Autodesk Fusion 360 part; units mm, degrees
(part 7 of 9)
sketch "Sketch13" plane through (0, 0.6, 0) normal (0, -1, 0) x (1, 0, 0)
  circle A0 centre (32.525, 66.675) radius 2
  circle A1 centre (245.269, 9.525) radius 2
  circle A2 centre (47.625, 9.525) radius 2
  circle A3 centre (220.025, 66.675) radius 2
  circle A4 centre (128.588, 37.025) radius 2
  arc A5 (94.0125, 35.575) -> (93.0125, 34.575) centre (94.0125, 34.575) ccw
  line L0 (94.0125, 35.575) -> (106.0125, 35.575)
  arc A6 (107.0125, 34.575) -> (106.0125, 35.575) centre (106.0125, 34.575) ccw
  line L1 (107.0125, 34.575) -> (107.0125, 22.575)
  arc A7 (106.0125, 21.575) -> (107.0125, 22.575) centre (106.0125, 22.575) ccw
  line L2 (106.0125, 21.575) -> (94.0125, 21.575)
  arc A8 (93.0125, 22.575) -> (94.0125, 21.575) centre (94.0125, 22.575) ccw
  line L3 (93.0125, 22.575) -> (93.0125, 34.575)
  arc A9 (132.1125, 35.575) -> (131.1125, 34.575) centre (132.1125, 34.575) ccw
  line L4 (132.1125, 35.575) -> (144.1125, 35.575)
  arc A10 (145.1125, 34.575) -> (144.1125, 35.575) centre (144.1125, 34.575) ccw
  line L5 (145.1125, 34.575) -> (145.1125, 22.575)
  arc A11 (144.1125, 21.575) -> (145.1125, 22.575) centre (144.1125, 22.575) ccw
  line L6 (144.1125, 21.575) -> (132.1125, 21.575)
  arc A12 (131.1125, 22.575) -> (132.1125, 21.575) centre (132.1125, 22.575) ccw
  line L7 (131.1125, 22.575) -> (131.1125, 34.575)
  arc A13 (251.175, 16.525) -> (250.175, 15.525) centre (251.175, 15.525) ccw
  line L8 (251.175, 16.525) -> (263.175, 16.525)
  arc A14 (264.175, 15.525) -> (263.175, 16.525) centre (263.175, 15.525) ccw
  line L9 (264.175, 15.525) -> (264.175, 3.525)
  arc A15 (263.175, 2.525) -> (264.175, 3.525) centre (263.175, 3.525) ccw
  line L10 (263.175, 2.525) -> (251.175, 2.525)
  arc A16 (250.175, 3.525) -> (251.175, 2.525) centre (251.175, 3.525) ccw
  line L11 (250.175, 3.525) -> (250.175, 15.525)
  arc A17 (217.8375, 54.625) -> (216.8375, 53.625) centre (217.8375, 53.625) ccw
  line L12 (217.8375, 54.625) -> (229.8375, 54.625)
  arc A18 (230.8375, 53.625) -> (229.8375, 54.625) centre (229.8375, 53.625) ccw
  line L13 (230.8375, 53.625) -> (230.8375, 41.625)
  arc A19 (229.8375, 40.625) -> (230.8375, 41.625) centre (229.8375, 41.625) ccw
  line L14 (229.8375, 40.625) -> (217.8375, 40.625)
  arc A20 (216.8375, 41.625) -> (217.8375, 40.625) centre (217.8375, 41.625) ccw
  line L15 (216.8375, 41.625) -> (216.8375, 53.625)
  arc A21 (179.7375, 54.625) -> (178.7375, 53.625) centre (179.7375, 53.625) ccw
  line L16 (179.7375, 54.625) -> (191.7375, 54.625)
  arc A22 (192.7375, 53.625) -> (191.7375, 54.625) centre (191.7375, 53.625) ccw
  line L17 (192.7375, 53.625) -> (192.7375, 41.625)
  arc A23 (191.7375, 40.625) -> (192.7375, 41.625) centre (191.7375, 41.625) ccw
  line L18 (191.7375, 40.625) -> (179.7375, 40.625)
  arc A24 (178.7375, 41.625) -> (179.7375, 40.625) centre (179.7375, 41.625) ccw
  line L19 (178.7375, 41.625) -> (178.7375, 53.625)
  arc A25 (108.3, 16.525) -> (107.3, 15.525) centre (108.3, 15.525) ccw
  line L20 (108.3, 16.525) -> (120.3, 16.525)
  arc A26 (121.3, 15.525) -> (120.3, 16.525) centre (120.3, 15.525) ccw
  line L21 (121.3, 15.525) -> (121.3, 3.525)
  arc A27 (120.3, 2.525) -> (121.3, 3.525) centre (120.3, 3.525) ccw
  line L22 (120.3, 2.525) -> (108.3, 2.525)
  arc A28 (107.3, 3.525) -> (108.3, 2.525) centre (108.3, 3.525) ccw
  line L23 (107.3, 3.525) -> (107.3, 15.525)
  arc A29 (203.55, 16.525) -> (202.55, 15.525) centre (203.55, 15.525) ccw
  line L24 (203.55, 16.525) -> (215.55, 16.525)
  arc A30 (216.55, 15.525) -> (215.55, 16.525) centre (215.55, 15.525) ccw
  line L25 (216.55, 15.525) -> (216.55, 3.525)
  arc A31 (215.55, 2.525) -> (216.55, 3.525) centre (215.55, 3.525) ccw
  line L26 (215.55, 2.525) -> (203.55, 2.525)
  arc A32 (202.55, 3.525) -> (203.55, 2.525) centre (203.55, 3.525) ccw
  line L27 (202.55, 3.525) -> (202.55, 15.525)
  arc A33 (189.2625, 35.575) -> (188.2625, 34.575) centre (189.2625, 34.575) ccw
  line L28 (189.2625, 35.575) -> (201.2625, 35.575)
  arc A34 (202.2625, 34.575) -> (201.2625, 35.575) centre (201.2625, 34.575) ccw
  line L29 (202.2625, 34.575) -> (202.2625, 22.575)
  arc A35 (201.2625, 21.575) -> (202.2625, 22.575) centre (201.2625, 22.575) ccw
  line L30 (201.2625, 21.575) -> (189.2625, 21.575)
  arc A36 (188.2625, 22.575) -> (189.2625, 21.575) centre (189.2625, 22.575) ccw
  line L31 (188.2625, 22.575) -> (188.2625, 34.575)
  arc A37 (146.4, 16.525) -> (145.4, 15.525) centre (146.4, 15.525) ccw
  line L32 (146.4, 16.525) -> (158.4, 16.525)
  arc A38 (159.4, 15.525) -> (158.4, 16.525) centre (158.4, 15.525) ccw
  line L33 (159.4, 15.525) -> (159.4, 3.525)
  arc A39 (158.4, 2.525) -> (159.4, 3.525) centre (158.4, 3.525) ccw
  line L34 (158.4, 2.525) -> (146.4, 2.525)
  arc A40 (145.4, 3.525) -> (146.4, 2.525) centre (146.4, 3.525) ccw
  line L35 (145.4, 3.525) -> (145.4, 15.525)
  arc A41 (113.0625, 35.575) -> (112.0625, 34.575) centre (113.0625, 34.575) ccw
  line L36 (113.0625, 35.575) -> (125.0625, 35.575)
  arc A42 (126.0625, 34.575) -> (125.0625, 35.575) centre (125.0625, 34.575) ccw
  line L37 (126.0625, 34.575) -> (126.0625, 22.575)
  arc A43 (125.0625, 21.575) -> (126.0625, 22.575) centre (125.0625, 22.575) ccw
  line L38 (125.0625, 21.575) -> (113.0625, 21.575)
  arc A44 (112.0625, 22.575) -> (113.0625, 21.575) centre (113.0625, 22.575) ccw
  line L39 (112.0625, 22.575) -> (112.0625, 34.575)
  arc A45 (127.35, 16.525) -> (126.35, 15.525) centre (127.35, 15.525) ccw
  line L40 (127.35, 16.525) -> (139.35, 16.525)
  arc A46 (140.35, 15.525) -> (139.35, 16.525) centre (139.35, 15.525) ccw
  line L41 (140.35, 15.525) -> (140.35, 3.525)
  arc A47 (139.35, 2.525) -> (140.35, 3.525) centre (139.35, 3.525) ccw
  line L42 (139.35, 2.525) -> (127.35, 2.525)
  arc A48 (126.35, 3.525) -> (127.35, 2.525) centre (127.35, 3.525) ccw
  line L43 (126.35, 3.525) -> (126.35, 15.525)
  arc A49 (170.2125, 35.575) -> (169.2125, 34.575) centre (170.2125, 34.575) ccw
  line L44 (170.2125, 35.575) -> (182.2125, 35.575)
  arc A50 (183.2125, 34.575) -> (182.2125, 35.575) centre (182.2125, 34.575) ccw
  line L45 (183.2125, 34.575) -> (183.2125, 22.575)
  arc A51 (182.2125, 21.575) -> (183.2125, 22.575) centre (182.2125, 22.575) ccw
  line L46 (182.2125, 21.575) -> (170.2125, 21.575)
  arc A52 (169.2125, 22.575) -> (170.2125, 21.575) centre (170.2125, 22.575) ccw
  line L47 (169.2125, 22.575) -> (169.2125, 34.575)
  arc A53 (224.9813, 73.675) -> (223.9813, 72.675) centre (224.9813, 72.675) ccw
  line L48 (224.9813, 73.675) -> (236.9813, 73.675)
  arc A54 (237.9812, 72.675) -> (236.9813, 73.675) centre (236.9813, 72.675) ccw
  line L49 (237.9812, 72.675) -> (237.9813, 60.675)
  arc A55 (236.9813, 59.675) -> (237.9813, 60.675) centre (236.9813, 60.675) ccw
  line L50 (236.9813, 59.675) -> (224.9813, 59.675)
  arc A56 (223.9812, 60.675) -> (224.9813, 59.675) centre (224.9813, 60.675) ccw
  line L51 (223.9812, 60.675) -> (223.9813, 72.675)
  arc A57 (198.7875, 54.625) -> (197.7875, 53.625) centre (198.7875, 53.625) ccw
  line L52 (198.7875, 54.625) -> (210.7875, 54.625)
  arc A58 (211.7875, 53.625) -> (210.7875, 54.625) centre (210.7875, 53.625) ccw
  line L53 (211.7875, 53.625) -> (211.7875, 41.625)
  arc A59 (210.7875, 40.625) -> (211.7875, 41.625) centre (210.7875, 41.625) ccw
  line L54 (210.7875, 40.625) -> (198.7875, 40.625)
  arc A60 (197.7875, 41.625) -> (198.7875, 40.625) centre (198.7875, 41.625) ccw
  line L55 (197.7875, 41.625) -> (197.7875, 53.625)
  arc A61 (51.15, 16.525) -> (50.15, 15.525) centre (51.15, 15.525) ccw
  line L56 (51.15, 16.525) -> (63.15, 16.525)
  arc A62 (64.15, 15.525) -> (63.15, 16.525) centre (63.15, 15.525) ccw
  line L57 (64.15, 15.525) -> (64.15, 3.525)
  arc A63 (63.15, 2.525) -> (64.15, 3.525) centre (63.15, 3.525) ccw
  line L58 (63.15, 2.525) -> (51.15, 2.525)
  arc A64 (50.15, 3.525) -> (51.15, 2.525) centre (51.15, 3.525) ccw
  line L59 (50.15, 3.525) -> (50.15, 15.525)
  arc A65 (8.2875, 16.525) -> (7.2875, 15.525) centre (8.2875, 15.525) ccw
  line L60 (8.2875, 16.525) -> (20.2875, 16.525)
  arc A66 (21.2875, 15.525) -> (20.2875, 16.525) centre (20.2875, 15.525) ccw
  line L61 (21.2875, 15.525) -> (21.2875, 3.525)
  arc A67 (20.2875, 2.525) -> (21.2875, 3.525) centre (20.2875, 3.525) ccw
  line L62 (20.2875, 2.525) -> (8.2875, 2.525)
  arc A68 (7.2875, 3.525) -> (8.2875, 2.525) centre (8.2875, 3.525) ccw
  line L63 (7.2875, 3.525) -> (7.2875, 15.525)
  arc A69 (208.3125, 35.575) -> (207.3125, 34.575) centre (208.3125, 34.575) ccw
  line L64 (208.3125, 35.575) -> (220.3125, 35.575)
  arc A70 (221.3125, 34.575) -> (220.3125, 35.575) centre (220.3125, 34.575) ccw
  line L65 (221.3125, 34.575) -> (221.3125, 22.575)
  arc A71 (220.3125, 21.575) -> (221.3125, 22.575) centre (220.3125, 22.575) ccw
  line L66 (220.3125, 21.575) -> (208.3125, 21.575)
  arc A72 (207.3125, 22.575) -> (208.3125, 21.575) centre (208.3125, 22.575) ccw
  line L67 (207.3125, 22.575) -> (207.3125, 34.575)
  arc A73 (227.3625, 16.525) -> (226.3625, 15.525) centre (227.3625, 15.525) ccw
  line L68 (227.3625, 16.525) -> (239.3625, 16.525)
  arc A74 (240.3625, 15.525) -> (239.3625, 16.525) centre (239.3625, 15.525) ccw
  line L69 (240.3625, 15.525) -> (240.3625, 3.525)
  arc A75 (239.3625, 2.525) -> (240.3625, 3.525) centre (239.3625, 3.525) ccw
  line L70 (239.3625, 2.525) -> (227.3625, 2.525)
  arc A76 (226.3625, 3.525) -> (227.3625, 2.525) centre (227.3625, 3.525) ccw
  line L71 (226.3625, 3.525) -> (226.3625, 15.525)
  arc A77 (74.9625, 35.575) -> (73.9625, 34.575) centre (74.9625, 34.575) ccw
  line L72 (74.9625, 35.575) -> (86.9625, 35.575)
  arc A78 (87.9625, 34.575) -> (86.9625, 35.575) centre (86.9625, 34.575) ccw
  line L73 (87.9625, 34.575) -> (87.9625, 22.575)
  arc A79 (86.9625, 21.575) -> (87.9625, 22.575) centre (86.9625, 22.575) ccw
  line L74 (86.9625, 21.575) -> (74.9625, 21.575)
  arc A80 (73.9625, 22.575) -> (74.9625, 21.575) centre (74.9625, 22.575) ccw
  line L75 (73.9625, 22.575) -> (73.9625, 34.575)
  arc A81 (41.625, 73.675) -> (40.625, 72.675) centre (41.625, 72.675) ccw
  line L76 (41.625, 73.675) -> (53.625, 73.675)
  arc A82 (54.625, 72.675) -> (53.625, 73.675) centre (53.625, 72.675) ccw
  line L77 (54.625, 72.675) -> (54.625, 60.675)
  arc A83 (53.625, 59.675) -> (54.625, 60.675) centre (53.625, 60.675) ccw
  line L78 (53.625, 59.675) -> (41.625, 59.675)
  arc A84 (40.625, 60.675) -> (41.625, 59.675) centre (41.625, 60.675) ccw
  line L79 (40.625, 60.675) -> (40.625, 72.675)
  arc A85 (89.25, 16.525) -> (88.25, 15.525) centre (89.25, 15.525) ccw
  line L80 (89.25, 16.525) -> (101.25, 16.525)
  arc A86 (102.25, 15.525) -> (101.25, 16.525) centre (101.25, 15.525) ccw
  line L81 (102.25, 15.525) -> (102.25, 3.525)
  arc A87 (101.25, 2.525) -> (102.25, 3.525) centre (101.25, 3.525) ccw
  line L82 (101.25, 2.525) -> (89.25, 2.525)
  arc A88 (88.25, 3.525) -> (89.25, 2.525) centre (89.25, 3.525) ccw
  line L83 (88.25, 3.525) -> (88.25, 15.525)
  arc A89 (151.1625, 35.575) -> (150.1625, 34.575) centre (151.1625, 34.575) ccw
  line L84 (151.1625, 35.575) -> (163.1625, 35.575)
  arc A90 (164.1625, 34.575) -> (163.1625, 35.575) centre (163.1625, 34.575) ccw
  line L85 (164.1625, 34.575) -> (164.1625, 22.575)
  arc A91 (163.1625, 21.575) -> (164.1625, 22.575) centre (163.1625, 22.575) ccw
  line L86 (163.1625, 21.575) -> (151.1625, 21.575)
  arc A92 (150.1625, 22.575) -> (151.1625, 21.575) centre (151.1625, 22.575) ccw
  line L87 (150.1625, 22.575) -> (150.1625, 34.575)
  arc A93 (172.5938, 73.675) -> (171.5938, 72.675) centre (172.5938, 72.675) ccw
  line L88 (172.5938, 73.675) -> (184.5938, 73.675)
  arc A94 (185.5937, 72.675) -> (184.5938, 73.675) centre (184.5937, 72.675) ccw
  line L89 (185.5937, 72.675) -> (185.5937, 60.675)
  arc A95 (184.5938, 59.675) -> (185.5937, 60.675) centre (184.5938, 60.675) ccw
  line L90 (184.5938, 59.675) -> (172.5937, 59.675)
  arc A96 (171.5938, 60.675) -> (172.5938, 59.675) centre (172.5938, 60.675) ccw
  line L91 (171.5937, 60.675) -> (171.5938, 72.675)
  arc A97 (70.2, 16.525) -> (69.2, 15.525) centre (70.2, 15.525) ccw
  line L92 (70.2, 16.525) -> (82.2, 16.525)
  arc A98 (83.2, 15.525) -> (82.2, 16.525) centre (82.2, 15.525) ccw
  line L93 (83.2, 15.525) -> (83.2, 3.525)
  arc A99 (82.2, 2.525) -> (83.2, 3.525) centre (82.2, 3.525) ccw
  line L94 (82.2, 2.525) -> (70.2, 2.525)
  arc A100 (69.2, 3.525) -> (70.2, 2.525) centre (70.2, 3.525) ccw
  line L95 (69.2, 3.525) -> (69.2, 15.525)
  arc A101 (46.3875, 54.625) -> (45.3875, 53.625) centre (46.3875, 53.625) ccw
  line L96 (46.3875, 54.625) -> (58.3875, 54.625)
  arc A102 (59.3875, 53.625) -> (58.3875, 54.625) centre (58.3875, 53.625) ccw
  line L97 (59.3875, 53.625) -> (59.3875, 41.625)
  arc A103 (58.3875, 40.625) -> (59.3875, 41.625) centre (58.3875, 41.625) ccw
  line L98 (58.3875, 40.625) -> (46.3875, 40.625)
  arc A104 (45.3875, 41.625) -> (46.3875, 40.625) centre (46.3875, 41.625) ccw
  line L99 (45.3875, 41.625) -> (45.3875, 53.625)
  arc A105 (55.9125, 35.575) -> (54.9125, 34.575) centre (55.9125, 34.575) ccw
  line L100 (55.9125, 35.575) -> (67.9125, 35.575)
  arc A106 (68.9125, 34.575) -> (67.9125, 35.575) centre (67.9125, 34.575) ccw
  line L101 (68.9125, 34.575) -> (68.9125, 22.575)
  arc A107 (67.9125, 21.575) -> (68.9125, 22.575) centre (67.9125, 22.575) ccw
  line L102 (67.9125, 21.575) -> (55.9125, 21.575)
  arc A108 (54.9125, 22.575) -> (55.9125, 21.575) centre (55.9125, 22.575) ccw
  line L103 (54.9125, 22.575) -> (54.9125, 34.575)
  arc A109 (45.1, 15.525) -> (44.1, 16.525) centre (44.1, 15.525) ccw
  line L104 (45.1, 15.525) -> (45.1, 3.525)
  arc A110 (44.1, 2.525) -> (45.1, 3.525) centre (44.1, 3.525) ccw
  line L105 (44.1, 2.525) -> (32.1, 2.525)
  arc A111 (31.1, 3.525) -> (32.1, 2.525) centre (32.1, 3.525) ccw
  line L106 (31.1, 3.525) -> (31.1, 15.525)
  arc A112 (32.1, 16.525) -> (31.1, 15.525) centre (32.1, 15.525) ccw
  line L107 (32.1, 16.525) -> (44.1, 16.525)
  arc A113 (184.5, 16.525) -> (183.5, 15.525) centre (184.5, 15.525) ccw
  line L108 (184.5, 16.525) -> (196.5, 16.525)
  arc A114 (197.5, 15.525) -> (196.5, 16.525) centre (196.5, 15.525) ccw
  line L109 (197.5, 15.525) -> (197.5, 3.525)
  arc A115 (196.5, 2.525) -> (197.5, 3.525) centre (196.5, 3.525) ccw
  line L110 (196.5, 2.525) -> (184.5, 2.525)
  arc A116 (183.5, 3.525) -> (184.5, 2.525) centre (184.5, 3.525) ccw
  line L111 (183.5, 3.525) -> (183.5, 15.525)
  arc A117 (261.3688, 34.575) -> (260.3688, 35.575) centre (260.3688, 34.575) ccw
  line L112 (261.3688, 34.575) -> (261.3688, 22.575)
  arc A118 (260.3688, 21.575) -> (261.3688, 22.575) centre (260.3688, 22.575) ccw
  line L113 (260.3688, 21.575) -> (230.1688, 21.575)
  arc A119 (229.1688, 22.575) -> (230.1688, 21.575) centre (230.1688, 22.575) ccw
  line L114 (229.1688, 22.575) -> (229.1688, 34.575)
  arc A120 (230.1688, 35.575) -> (229.1688, 34.575) centre (230.1688, 34.575) ccw
  line L115 (230.1688, 35.575) -> (260.3688, 35.575)
  arc A121 (67.8188, 73.675) -> (66.8188, 72.675) centre (67.8188, 72.675) ccw
  line L116 (67.8188, 73.675) -> (79.8188, 73.675)
  arc A122 (80.8188, 72.675) -> (79.8188, 73.675) centre (79.8188, 72.675) ccw
  line L117 (80.8187, 72.675) -> (80.8187, 60.675)
  arc A123 (79.8188, 59.675) -> (80.8188, 60.675) centre (79.8188, 60.675) ccw
  line L118 (79.8188, 59.675) -> (67.8188, 59.675)
  arc A124 (66.8188, 60.675) -> (67.8188, 59.675) centre (67.8188, 60.675) ccw
  line L119 (66.8188, 60.675) -> (66.8188, 72.675)
  arc A125 (165.45, 16.525) -> (164.45, 15.525) centre (165.45, 15.525) ccw
  line L120 (165.45, 16.525) -> (177.45, 16.525)
  arc A126 (178.45, 15.525) -> (177.45, 16.525) centre (177.45, 15.525) ccw
  line L121 (178.45, 15.525) -> (178.45, 3.525)
  arc A127 (177.45, 2.525) -> (178.45, 3.525) centre (177.45, 3.525) ccw
  line L122 (177.45, 2.525) -> (165.45, 2.525)
  arc A128 (164.45, 3.525) -> (165.45, 2.525) centre (165.45, 3.525) ccw
  line L123 (164.45, 3.525) -> (164.45, 15.525)
  arc A129 (14.4313, 60.675) -> (15.4313, 59.675) centre (15.4313, 60.675) ccw
  line L124 (14.4313, 60.675) -> (14.4313, 72.675)
  arc A130 (15.4313, 73.675) -> (14.4313, 72.675) centre (15.4313, 72.675) ccw
  line L125 (15.4313, 73.675) -> (27.4313, 73.675)
  arc A131 (28.4312, 72.675) -> (27.4313, 73.675) centre (27.4312, 72.675) ccw
  line L126 (28.4312, 72.675) -> (28.4313, 60.675)
  arc A132 (27.4313, 59.675) -> (28.4313, 60.675) centre (27.4313, 60.675) ccw
  line L127 (27.4313, 59.675) -> (15.4313, 59.675)
  arc A133 (244.0312, 54.625) -> (243.0313, 53.625) centre (244.0312, 53.625) ccw
  line L128 (244.0312, 54.625) -> (256.0312, 54.625)
  arc A134 (257.0312, 53.625) -> (256.0312, 54.625) centre (256.0312, 53.625) ccw
  line L129 (257.0312, 53.625) -> (257.0312, 41.625)
  arc A135 (256.0312, 40.625) -> (257.0312, 41.625) centre (256.0312, 41.625) ccw
  line L130 (256.0312, 40.625) -> (244.0312, 40.625)
  arc A136 (243.0313, 41.625) -> (244.0312, 40.625) centre (244.0312, 41.625) ccw
  line L131 (243.0312, 41.625) -> (243.0312, 53.625)
  arc A137 (198.7875, 73.675) -> (197.7875, 72.675) centre (198.7875, 72.675) ccw
  line L132 (198.7875, 73.675) -> (210.7875, 73.675)
  arc A138 (211.7875, 72.675) -> (210.7875, 73.675) centre (210.7875, 72.675) ccw
  line L133 (211.7875, 72.675) -> (211.7875, 60.675)
  arc A139 (210.7875, 59.675) -> (211.7875, 60.675) centre (210.7875, 60.675) ccw
  line L134 (210.7875, 59.675) -> (198.7875, 59.675)
  arc A140 (197.7875, 60.675) -> (198.7875, 59.675) centre (198.7875, 60.675) ccw
  line L135 (197.7875, 60.675) -> (197.7875, 72.675)
  arc A141 (65.4375, 54.625) -> (64.4375, 53.625) centre (65.4375, 53.625) ccw
  line L136 (65.4375, 54.625) -> (77.4375, 54.625)
  arc A142 (78.4375, 53.625) -> (77.4375, 54.625) centre (77.4375, 53.625) ccw
  line L137 (78.4375, 53.625) -> (78.4375, 41.625)
  arc A143 (77.4375, 40.625) -> (78.4375, 41.625) centre (77.4375, 41.625) ccw
  line L138 (77.4375, 40.625) -> (65.4375, 40.625)
  arc A144 (64.4375, 41.625) -> (65.4375, 40.625) centre (65.4375, 41.625) ccw
  line L139 (64.4375, 41.625) -> (64.4375, 53.625)
  arc A145 (35.8625, 34.575) -> (34.8625, 35.575) centre (34.8625, 34.575) ccw
  line L140 (34.8625, 35.575) -> (24.6688, 35.575)
  arc A146 (24.6688, 35.575) -> (23.6687, 34.575) centre (24.6688, 34.575) ccw
  line L141 (23.6687, 34.575) -> (23.6688, 22.575)
  arc A147 (22.6687, 21.575) -> (23.6688, 22.575) centre (22.6688, 22.575) ccw
  line L142 (22.6687, 21.575) -> (10.6688, 21.575)
  arc A148 (9.6687, 22.575) -> (10.6688, 21.575) centre (10.6687, 22.575) ccw
  line L143 (9.6687, 22.575) -> (9.6687, 34.575)
  arc A149 (9.6687, 34.575) -> (8.6687, 35.575) centre (8.6687, 34.575) ccw
  line L144 (8.6687, 35.575) -> (4.3312, 35.575)
  line L145 (4.3312, 35.575) -> (4.3313, 39.625)
  arc A150 (5.3312, 40.625) -> (4.3312, 39.625) centre (5.3312, 39.625) ccw
  line L146 (5.3312, 40.625) -> (5.3312, 55.625)
  line L147 (5.3312, 55.625) -> (3, 55.625)
  arc A151 (3, 55.625) -> (1.525, 54.15) centre (3, 54.15) ccw
  line L148 (1.525, 54.15) -> (1.525, 3)
  arc A152 (1.525, 3) -> (3, 1.525) centre (3, 3) ccw
  line L149 (3, 1.525) -> (263.7, 1.525)
  arc A153 (263.7, 1.525) -> (265.175, 3) centre (263.7, 3) ccw
  line L150 (265.175, 3) -> (265.175, 54.15)
  arc A154 (265.175, 54.15) -> (263.7, 55.625) centre (263.7, 54.15) ccw
  line L151 (263.7, 55.625) -> (243.8875, 55.625)
  arc A155 (241.3625, 58.15) -> (243.8875, 55.625) centre (243.8875, 58.15) ccw
  line L152 (241.3625, 58.15) -> (241.3625, 73.2)
  arc A156 (241.3625, 73.2) -> (239.8875, 74.675) centre (239.8875, 73.2) ccw
  line L153 (239.8875, 74.675) -> (163.7375, 74.675)
  line L154 (163.7375, 74.675) -> (163.7375, 59.675)
  arc A157 (164.7375, 58.675) -> (163.7375, 59.675) centre (163.7375, 58.675) ccw
  line L155 (164.7375, 58.675) -> (164.7375, 55.625)
  line L156 (164.7375, 55.625) -> (168.1875, 55.625)
  arc A158 (169.1875, 54.625) -> (168.1875, 55.625) centre (168.1875, 54.625) ccw
  line L157 (169.1875, 54.625) -> (172.6875, 54.625)
  arc A159 (173.6875, 53.625) -> (172.6875, 54.625) centre (172.6875, 53.625) ccw
  line L158 (173.6875, 53.625) -> (173.6875, 41.625)
  arc A160 (172.6875, 40.625) -> (173.6875, 41.625) centre (172.6875, 41.625) ccw
  line L159 (172.6875, 40.625) -> (160.6875, 40.625)
  arc A161 (159.6875, 41.625) -> (160.6875, 40.625) centre (160.6875, 41.625) ccw
  line L160 (159.6875, 41.625) -> (159.6875, 53.625)
  arc A162 (159.6875, 53.625) -> (158.6875, 54.625) centre (158.6875, 53.625) ccw
  line L161 (158.6875, 54.625) -> (155.6375, 54.625)
  arc A163 (155.6375, 54.625) -> (154.6375, 53.625) centre (155.6375, 53.625) ccw
  line L162 (154.6375, 53.625) -> (154.6375, 41.625)
  arc A164 (153.6375, 40.625) -> (154.6375, 41.625) centre (153.6375, 41.625) ccw
  line L163 (153.6375, 40.625) -> (141.6375, 40.625)
  arc A165 (140.6375, 41.625) -> (141.6375, 40.625) centre (141.6375, 41.625) ccw
  line L164 (140.6375, 41.625) -> (140.6375, 53.625)
  arc A166 (140.6375, 53.625) -> (139.6375, 54.625) centre (139.6375, 53.625) ccw
  line L165 (139.6375, 54.625) -> (136.5875, 54.625)
  arc A167 (136.5875, 54.625) -> (135.5875, 53.625) centre (136.5875, 53.625) ccw
  line L166 (135.5875, 53.625) -> (135.5875, 41.625)
  arc A168 (134.5875, 40.625) -> (135.5875, 41.625) centre (134.5875, 41.625) ccw
  line L167 (134.5875, 40.625) -> (122.5875, 40.625)
  arc A169 (121.5875, 41.625) -> (122.5875, 40.625) centre (122.5875, 41.625) ccw
  line L168 (121.5875, 41.625) -> (121.5875, 53.625)
  arc A170 (121.5875, 53.625) -> (120.5875, 54.625) centre (120.5875, 53.625) ccw
  line L169 (120.5875, 54.625) -> (117.5375, 54.625)
  arc A171 (117.5375, 54.625) -> (116.5375, 53.625) centre (117.5375, 53.625) ccw
  line L170 (116.5375, 53.625) -> (116.5375, 41.625)
  arc A172 (115.5375, 40.625) -> (116.5375, 41.625) centre (115.5375, 41.625) ccw
  line L171 (115.5375, 40.625) -> (103.5375, 40.625)
  arc A173 (102.5375, 41.625) -> (103.5375, 40.625) centre (103.5375, 41.625) ccw
  line L172 (102.5375, 41.625) -> (102.5375, 53.625)
  arc A174 (102.5375, 53.625) -> (101.5375, 54.625) centre (101.5375, 53.625) ccw
  line L173 (101.5375, 54.625) -> (98.4875, 54.625)
  arc A175 (98.4875, 54.625) -> (97.4875, 53.625) centre (98.4875, 53.625) ccw
  line L174 (97.4875, 53.625) -> (97.4875, 41.625)
  arc A176 (96.4875, 40.625) -> (97.4875, 41.625) centre (96.4875, 41.625) ccw
  line L175 (96.4875, 40.625) -> (84.4875, 40.625)
  arc A177 (83.4875, 41.625) -> (84.4875, 40.625) centre (84.4875, 41.625) ccw
  line L176 (83.4875, 41.625) -> (83.4875, 53.625)
  arc A178 (84.4875, 54.625) -> (83.4875, 53.625) centre (84.4875, 53.625) ccw
  line L177 (84.4875, 54.625) -> (87.9875, 54.625)
  arc A179 (88.9875, 55.625) -> (87.9875, 54.625) centre (88.9875, 54.625) ccw
  line L178 (88.9875, 55.625) -> (90.0563, 55.625)
  line L179 (90.0563, 55.625) -> (90.0563, 58.675)
  arc A180 (91.0563, 59.675) -> (90.0563, 58.675) centre (91.0563, 58.675) ccw
  line L180 (91.0563, 59.675) -> (91.0563, 74.675)
  line L181 (91.0563, 74.675) -> (12.525, 74.675)
  arc A181 (12.525, 74.675) -> (11.05, 73.2) centre (12.525, 73.2) ccw
  line L182 (11.05, 73.2) -> (11.05, 58.15)
  arc A182 (10.5375, 56.625) -> (11.05, 58.15) centre (8.525, 58.15) ccw
  line L183 (10.5375, 56.625) -> (12.3312, 56.625)
  arc A183 (13.3312, 55.625) -> (12.3312, 56.625) centre (12.3312, 55.625) ccw
  line L184 (13.3312, 55.625) -> (13.3312, 54.625)
  line L185 (13.3312, 54.625) -> (18.9313, 54.625)
  arc A184 (19.9313, 55.625) -> (18.9313, 54.625) centre (19.9313, 54.625) ccw
  line L186 (19.9313, 55.625) -> (22.9313, 55.625)
  arc A185 (23.9313, 54.625) -> (22.9313, 55.625) centre (22.9313, 54.625) ccw
  line L187 (23.9313, 54.625) -> (29.5312, 54.625)
  line L188 (29.5312, 54.625) -> (29.5312, 55.625)
  arc A186 (30.5312, 56.625) -> (29.5312, 55.625) centre (30.5312, 55.625) ccw
  line L189 (30.5312, 56.625) -> (36.5312, 56.625)
  arc A187 (37.5312, 55.625) -> (36.5312, 56.625) centre (36.5312, 55.625) ccw
  line L190 (37.5312, 55.625) -> (37.5312, 40.625)
  arc A188 (38.5312, 39.625) -> (37.5312, 40.625) centre (37.5312, 39.625) ccw
  line L191 (38.5312, 39.625) -> (38.5312, 36.575)
  line L192 (38.5312, 36.575) -> (44.3625, 36.575)
  arc A189 (45.3625, 35.575) -> (44.3625, 36.575) centre (44.3625, 35.575) ccw
  line L193 (45.3625, 35.575) -> (48.8625, 35.575)
  arc A190 (49.8625, 34.575) -> (48.8625, 35.575) centre (48.8625, 34.575) ccw
  line L194 (49.8625, 34.575) -> (49.8625, 22.575)
  arc A191 (48.8625, 21.575) -> (49.8625, 22.575) centre (48.8625, 22.575) ccw
  line L195 (48.8625, 21.575) -> (36.8625, 21.575)
  arc A192 (35.8625, 22.575) -> (36.8625, 21.575) centre (36.8625, 22.575) ccw
  line L196 (35.8625, 22.575) -> (35.8625, 34.575)
  line L197 (229.1688, 31.8208) -> (237.1688, 31.8208)
  line L198 (237.1688, 31.8208) -> (237.1688, 36.575)
  line L199 (236.1688, 37.575) -> (230.1688, 37.575)
  line L200 (229.1688, 36.575) -> (229.1688, 31.8208)
  line L201 (261.3688, 33.0848) -> (253.3688, 33.0848)
  line L202 (253.3688, 33.0848) -> (253.3688, 36.575)
  line L203 (254.3688, 37.575) -> (260.3688, 37.575)
  line L204 (261.3688, 36.575) -> (261.3688, 33.0848)
  line L205 (242.7688, 35.575) -> (247.7688, 35.575)
  line L206 (247.7688, 35.575) -> (247.7688, 36.575)
  line L207 (247.7688, 36.575) -> (242.7688, 36.575)
  line L208 (242.7688, 36.575) -> (242.7688, 35.575)
  arc A193 (230.1688, 37.575) -> (229.1688, 36.575) centre (230.1688, 36.575) ccw
  arc A194 (237.1688, 36.575) -> (236.1688, 37.575) centre (236.1687, 36.575) ccw
  arc A195 (254.3688, 37.575) -> (253.3688, 36.575) centre (254.3688, 36.575) ccw
  arc A196 (261.3688, 36.575) -> (260.3688, 37.575) centre (260.3688, 36.575) ccw
  line L209 (262.3688, 16.525) -> (262.3688, 21.5664)
  line L210 (261.3688, 22.5664) -> (229.1688, 22.5664)
  line L211 (228.1688, 21.5664) -> (228.1688, 16.525)
  line L212 (240.3625, 12.8505) -> (250.175, 12.8505)
  line L213 (250.175, 12.8505) -> (250.175, 15.525)
  line L214 (249.175, 16.525) -> (241.3625, 16.525)
  line L215 (240.3625, 15.525) -> (240.3625, 12.8505)
  arc A197 (241.3625, 16.525) -> (240.3625, 15.525) centre (241.3625, 15.525) ccw
  arc A198 (250.175, 15.525) -> (249.175, 16.525) centre (249.175, 15.525) ccw
  line L216 (228.1688, 16.525) -> (239.3625, 16.525)
  line L217 (241.3625, 16.525) -> (249.175, 16.525)
  line L218 (251.175, 16.525) -> (262.3688, 16.525)
  arc A199 (229.1688, 22.5664) -> (228.1688, 21.5664) centre (229.1688, 21.5664) ccw
  arc A200 (262.3688, 21.5664) -> (261.3688, 22.5664) centre (261.3688, 21.5664) ccw
  dimension "d192" = 8
  dimension "d193" = 8
  dimension "d194" = 2
  dimension "d195" = 2
  dimension "d196" = 5
  dimension "d197" = 1
  dimension "d198" = 13.6
  dimension "d199" = 1
  dimension "d200" = 1
  dimension "d201" = 1
  dimension "d202" = 1
  dimension "d203" = 1
  constraint horizontal L197
  constraint vertical L198
  constraint horizontal L199
  constraint vertical L200
  constraint coincident L114 L197.start
  constraint horizontal L201
  constraint vertical L202
  constraint horizontal L203
  constraint vertical L204
  constraint coincident L112 L201.start
  constraint horizontal L205
  constraint vertical L206
  constraint horizontal L207
  constraint vertical L208
  constraint coincident L115 L205.start
  constraint tangent L199 A193
  constraint tangent L200 A193
  constraint tangent L198 A194
  constraint tangent L199 A194
  constraint equal A193 A194
  constraint tangent L202 A195
  constraint tangent L203 A195
  constraint equal A193 A195
  constraint tangent L203 A196
  constraint tangent L204 A196
  constraint equal A193 A196
  constraint horizontal L216
  constraint vertical L209
  constraint horizontal L210
  constraint vertical L211
  constraint coincident L68 L211.end
  constraint horizontal L212
  constraint vertical L213
  constraint horizontal L214
  constraint vertical L215
  constraint coincident L69 L212.start
  constraint tangent L214 A197
  constraint tangent L215 A197
  constraint tangent L213 A198
  constraint tangent L214 A198
  constraint equal A197 A198
  constraint collinear L216 L217
  constraint collinear L217 L218
  constraint tangent L210 A199
  constraint tangent L211 A199
  constraint tangent L209 A200
  constraint tangent L210 A200
  constraint equal A199 A200
  measures "d192" distance of L197.start L197.end
  measures "d193" distance of L201.start L201.end
  measures "d194" distance of L115 L203
  measures "d195" distance of L115 L199
  measures "d196" distance of L205.start L205.end
  measures "d197" distance of L205.start L207.end
  measures "d198" distance of L112 L205.end
  measures "d199" radius of A193
  measures "d200" distance of L112 L209
  measures "d201" distance of L114 L211
  measures "d202" radius of A197
  measures "d203" radius of A199
extrude "Extrude12" cut sketch "Sketch13" against normal blind 3 contours A13 L8 L68 A74 A118 L113 A119 L209 L211 L214 A197 A198 L216 L217 L218 A199 A200 | A117 L115 L202 L203 L204 A195 A196 | A120 L115 L198 L199 L200 A193 A194 | L115 L205 L206 L207 L208
fillet "Fillet9" radius 1 1 edges at (242.7688, 2.1, 36.575)
fillet "Fillet10" radius 1 1 edges at (247.7688, 2.1, 36.575)
sketch "Sketch14" plane through (0, 0.6, 0) normal (0, -1, 0) x (1, 0, 0)
  arc A0 (35.8625, 34.575) -> (34.8625, 35.575) centre (34.8625, 34.575) ccw
  line L0 (34.8625, 35.575) -> (24.6688, 35.575)
  arc A1 (24.6688, 35.575) -> (23.6687, 34.575) centre (24.6688, 34.575) ccw
  line L1 (23.6687, 34.575) -> (23.6688, 22.575)
  arc A2 (22.6687, 21.575) -> (23.6688, 22.575) centre (22.6688, 22.575) ccw
  line L2 (22.6687, 21.575) -> (10.6688, 21.575)
  arc A3 (9.6687, 22.575) -> (10.6688, 21.575) centre (10.6687, 22.575) ccw
  line L3 (9.6687, 22.575) -> (9.6687, 34.575)
  arc A4 (9.6687, 34.575) -> (8.6687, 35.575) centre (8.6687, 34.575) ccw
  line L4 (8.6687, 35.575) -> (4.3312, 35.575)
  line L5 (4.3312, 35.575) -> (4.3313, 39.625)
  arc A5 (5.3312, 40.625) -> (4.3312, 39.625) centre (5.3312, 39.625) ccw
  line L6 (5.3312, 40.625) -> (5.3312, 55.625)
  line L7 (5.3312, 55.625) -> (3, 55.625)
  arc A6 (3, 55.625) -> (1.525, 54.15) centre (3, 54.15) ccw
  line L8 (1.525, 54.15) -> (1.525, 3)
  arc A7 (1.525, 3) -> (3, 1.525) centre (3, 3) ccw
  line L9 (3, 1.525) -> (263.7, 1.525)
  arc A8 (263.7, 1.525) -> (265.175, 3) centre (263.7, 3) ccw
  line L10 (265.175, 3) -> (265.175, 54.15)
  arc A9 (265.175, 54.15) -> (263.7, 55.625) centre (263.7, 54.15) ccw
  line L11 (263.7, 55.625) -> (243.8875, 55.625)
  arc A10 (241.3625, 58.15) -> (243.8875, 55.625) centre (243.8875, 58.15) ccw
  line L12 (241.3625, 58.15) -> (241.3625, 73.2)
  arc A11 (241.3625, 73.2) -> (239.8875, 74.675) centre (239.8875, 73.2) ccw
  line L13 (239.8875, 74.675) -> (163.7375, 74.675)
  line L14 (163.7375, 74.675) -> (163.7375, 59.675)
  arc A12 (164.7375, 58.675) -> (163.7375, 59.675) centre (163.7375, 58.675) ccw
  line L15 (164.7375, 58.675) -> (164.7375, 55.625)
  line L16 (164.7375, 55.625) -> (168.1875, 55.625)
  arc A13 (169.1875, 54.625) -> (168.1875, 55.625) centre (168.1875, 54.625) ccw
  line L17 (169.1875, 54.625) -> (172.6875, 54.625)
  arc A14 (173.6875, 53.625) -> (172.6875, 54.625) centre (172.6875, 53.625) ccw
  line L18 (173.6875, 53.625) -> (173.6875, 41.625)
  arc A15 (172.6875, 40.625) -> (173.6875, 41.625) centre (172.6875, 41.625) ccw
  line L19 (172.6875, 40.625) -> (160.6875, 40.625)
  arc A16 (159.6875, 41.625) -> (160.6875, 40.625) centre (160.6875, 41.625) ccw
  line L20 (159.6875, 41.625) -> (159.6875, 53.625)
  arc A17 (159.6875, 53.625) -> (158.6875, 54.625) centre (158.6875, 53.625) ccw
  line L21 (158.6875, 54.625) -> (155.6375, 54.625)
  arc A18 (155.6375, 54.625) -> (154.6375, 53.625) centre (155.6375, 53.625) ccw
  line L22 (154.6375, 53.625) -> (154.6375, 41.625)
  arc A19 (153.6375, 40.625) -> (154.6375, 41.625) centre (153.6375, 41.625) ccw
  line L23 (153.6375, 40.625) -> (141.6375, 40.625)
  arc A20 (140.6375, 41.625) -> (141.6375, 40.625) centre (141.6375, 41.625) ccw
  line L24 (140.6375, 41.625) -> (140.6375, 53.625)
  arc A21 (140.6375, 53.625) -> (139.6375, 54.625) centre (139.6375, 53.625) ccw
  line L25 (139.6375, 54.625) -> (136.5875, 54.625)
  arc A22 (136.5875, 54.625) -> (135.5875, 53.625) centre (136.5875, 53.625) ccw
  line L26 (135.5875, 53.625) -> (135.5875, 41.625)
  arc A23 (134.5875, 40.625) -> (135.5875, 41.625) centre (134.5875, 41.625) ccw
  line L27 (134.5875, 40.625) -> (122.5875, 40.625)
  arc A24 (121.5875, 41.625) -> (122.5875, 40.625) centre (122.5875, 41.625) ccw
  line L28 (121.5875, 41.625) -> (121.5875, 53.625)
  arc A25 (121.5875, 53.625) -> (120.5875, 54.625) centre (120.5875, 53.625) ccw
  line L29 (120.5875, 54.625) -> (117.5375, 54.625)
  arc A26 (117.5375, 54.625) -> (116.5375, 53.625) centre (117.5375, 53.625) ccw
  line L30 (116.5375, 53.625) -> (116.5375, 41.625)
  arc A27 (115.5375, 40.625) -> (116.5375, 41.625) centre (115.5375, 41.625) ccw
  line L31 (115.5375, 40.625) -> (103.5375, 40.625)
  arc A28 (102.5375, 41.625) -> (103.5375, 40.625) centre (103.5375, 41.625) ccw
  line L32 (102.5375, 41.625) -> (102.5375, 53.625)
  arc A29 (102.5375, 53.625) -> (101.5375, 54.625) centre (101.5375, 53.625) ccw
  line L33 (101.5375, 54.625) -> (98.4875, 54.625)
  arc A30 (98.4875, 54.625) -> (97.4875, 53.625) centre (98.4875, 53.625) ccw
  line L34 (97.4875, 53.625) -> (97.4875, 41.625)
  arc A31 (96.4875, 40.625) -> (97.4875, 41.625) centre (96.4875, 41.625) ccw
  line L35 (96.4875, 40.625) -> (84.4875, 40.625)
  arc A32 (83.4875, 41.625) -> (84.4875, 40.625) centre (84.4875, 41.625) ccw
  line L36 (83.4875, 41.625) -> (83.4875, 53.625)
  arc A33 (84.4875, 54.625) -> (83.4875, 53.625) centre (84.4875, 53.625) ccw
  line L37 (84.4875, 54.625) -> (87.9875, 54.625)
  arc A34 (88.9875, 55.625) -> (87.9875, 54.625) centre (88.9875, 54.625) ccw
  line L38 (88.9875, 55.625) -> (90.0563, 55.625)
  line L39 (90.0563, 55.625) -> (90.0563, 58.675)
  arc A35 (91.0563, 59.675) -> (90.0563, 58.675) centre (91.0563, 58.675) ccw
  line L40 (91.0563, 59.675) -> (91.0563, 74.675)
  line L41 (91.0563, 74.675) -> (12.525, 74.675)
  arc A36 (12.525, 74.675) -> (11.05, 73.2) centre (12.525, 73.2) ccw
  line L42 (11.05, 73.2) -> (11.05, 58.15)
  arc A37 (10.5375, 56.625) -> (11.05, 58.15) centre (8.525, 58.15) ccw
  line L43 (10.5375, 56.625) -> (12.3312, 56.625)
  arc A38 (13.3312, 55.625) -> (12.3312, 56.625) centre (12.3312, 55.625) ccw
  line L44 (13.3312, 55.625) -> (13.3312, 54.625)
  line L45 (13.3312, 54.625) -> (18.9313, 54.625)
  arc A39 (19.9313, 55.625) -> (18.9313, 54.625) centre (19.9313, 54.625) ccw
  line L46 (19.9313, 55.625) -> (22.9313, 55.625)
  arc A40 (23.9313, 54.625) -> (22.9313, 55.625) centre (22.9313, 54.625) ccw
  line L47 (23.9313, 54.625) -> (29.5312, 54.625)
  line L48 (29.5312, 54.625) -> (29.5312, 55.625)
  arc A41 (30.5312, 56.625) -> (29.5312, 55.625) centre (30.5312, 55.625) ccw
  line L49 (30.5312, 56.625) -> (36.5312, 56.625)
  arc A42 (37.5312, 55.625) -> (36.5312, 56.625) centre (36.5312, 55.625) ccw
  line L50 (37.5312, 55.625) -> (37.5312, 40.625)
  arc A43 (38.5312, 39.625) -> (37.5312, 40.625) centre (37.5312, 39.625) ccw
  line L51 (38.5312, 39.625) -> (38.5312, 36.575)
  line L52 (38.5312, 36.575) -> (44.3625, 36.575)
  arc A44 (45.3625, 35.575) -> (44.3625, 36.575) centre (44.3625, 35.575) ccw
  line L53 (45.3625, 35.575) -> (48.8625, 35.575)
  arc A45 (49.8625, 34.575) -> (48.8625, 35.575) centre (48.8625, 34.575) ccw
  line L54 (49.8625, 34.575) -> (49.8625, 22.575)
  arc A46 (48.8625, 21.575) -> (49.8625, 22.575) centre (48.8625, 22.575) ccw
  line L55 (48.8625, 21.575) -> (36.8625, 21.575)
  arc A47 (35.8625, 22.575) -> (36.8625, 21.575) centre (36.8625, 22.575) ccw
  line L56 (35.8625, 22.575) -> (35.8625, 34.575)
  arc A48 (65.4375, 54.625) -> (64.4375, 53.625) centre (65.4375, 53.625) ccw
  line L57 (65.4375, 54.625) -> (77.4375, 54.625)
  arc A49 (78.4375, 53.625) -> (77.4375, 54.625) centre (77.4375, 53.625) ccw
  line L58 (78.4375, 53.625) -> (78.4375, 41.625)
  arc A50 (77.4375, 40.625) -> (78.4375, 41.625) centre (77.4375, 41.625) ccw
  line L59 (77.4375, 40.625) -> (65.4375, 40.625)
  arc A51 (64.4375, 41.625) -> (65.4375, 40.625) centre (65.4375, 41.625) ccw
  line L60 (64.4375, 41.625) -> (64.4375, 53.625)
  arc A52 (198.7875, 73.675) -> (197.7875, 72.675) centre (198.7875, 72.675) ccw
  line L61 (198.7875, 73.675) -> (210.7875, 73.675)
  arc A53 (211.7875, 72.675) -> (210.7875, 73.675) centre (210.7875, 72.675) ccw
  line L62 (211.7875, 72.675) -> (211.7875, 60.675)
  arc A54 (210.7875, 59.675) -> (211.7875, 60.675) centre (210.7875, 60.675) ccw
  line L63 (210.7875, 59.675) -> (198.7875, 59.675)
  arc A55 (197.7875, 60.675) -> (198.7875, 59.675) centre (198.7875, 60.675) ccw
  line L64 (197.7875, 60.675) -> (197.7875, 72.675)
  arc A56 (244.0312, 54.625) -> (243.0313, 53.625) centre (244.0312, 53.625) ccw
  line L65 (244.0312, 54.625) -> (256.0312, 54.625)
  arc A57 (257.0312, 53.625) -> (256.0312, 54.625) centre (256.0312, 53.625) ccw
  line L66 (257.0312, 53.625) -> (257.0312, 41.625)
  arc A58 (256.0312, 40.625) -> (257.0312, 41.625) centre (256.0312, 41.625) ccw
  line L67 (256.0312, 40.625) -> (244.0312, 40.625)
  arc A59 (243.0313, 41.625) -> (244.0312, 40.625) centre (244.0312, 41.625) ccw
  line L68 (243.0312, 41.625) -> (243.0312, 53.625)
  arc A60 (14.4313, 60.675) -> (15.4313, 59.675) centre (15.4313, 60.675) ccw
  line L69 (14.4313, 60.675) -> (14.4313, 72.675)
  arc A61 (15.4313, 73.675) -> (14.4313, 72.675) centre (15.4313, 72.675) ccw
  line L70 (15.4313, 73.675) -> (27.4313, 73.675)
  arc A62 (28.4312, 72.675) -> (27.4313, 73.675) centre (27.4312, 72.675) ccw
  line L71 (28.4312, 72.675) -> (28.4313, 60.675)
  arc A63 (27.4313, 59.675) -> (28.4313, 60.675) centre (27.4313, 60.675) ccw
  line L72 (27.4313, 59.675) -> (15.4313, 59.675)
  arc A64 (165.45, 16.525) -> (164.45, 15.525) centre (165.45, 15.525) ccw
  line L73 (165.45, 16.525) -> (177.45, 16.525)
  arc A65 (178.45, 15.525) -> (177.45, 16.525) centre (177.45, 15.525) ccw
  line L74 (178.45, 15.525) -> (178.45, 3.525)
  arc A66 (177.45, 2.525) -> (178.45, 3.525) centre (177.45, 3.525) ccw
  line L75 (177.45, 2.525) -> (165.45, 2.525)
  arc A67 (164.45, 3.525) -> (165.45, 2.525) centre (165.45, 3.525) ccw
  line L76 (164.45, 3.525) -> (164.45, 15.525)
  arc A68 (67.8188, 73.675) -> (66.8188, 72.675) centre (67.8188, 72.675) ccw
  line L77 (67.8188, 73.675) -> (79.8188, 73.675)
  arc A69 (80.8188, 72.675) -> (79.8188, 73.675) centre (79.8188, 72.675) ccw
  line L78 (80.8187, 72.675) -> (80.8187, 60.675)
  arc A70 (79.8188, 59.675) -> (80.8188, 60.675) centre (79.8188, 60.675) ccw
  line L79 (79.8188, 59.675) -> (67.8188, 59.675)
  arc A71 (66.8188, 60.675) -> (67.8188, 59.675) centre (67.8188, 60.675) ccw
  line L80 (66.8188, 60.675) -> (66.8188, 72.675)
  arc A72 (184.5, 16.525) -> (183.5, 15.525) centre (184.5, 15.525) ccw
  line L81 (184.5, 16.525) -> (196.5, 16.525)
  arc A73 (197.5, 15.525) -> (196.5, 16.525) centre (196.5, 15.525) ccw
  line L82 (197.5, 15.525) -> (197.5, 3.525)
  arc A74 (196.5, 2.525) -> (197.5, 3.525) centre (196.5, 3.525) ccw
  line L83 (196.5, 2.525) -> (184.5, 2.525)
  arc A75 (183.5, 3.525) -> (184.5, 2.525) centre (184.5, 3.525) ccw
  line L84 (183.5, 3.525) -> (183.5, 15.525)
  arc A76 (45.1, 15.525) -> (44.1, 16.525) centre (44.1, 15.525) ccw
  line L85 (45.1, 15.525) -> (45.1, 3.525)
  arc A77 (44.1, 2.525) -> (45.1, 3.525) centre (44.1, 3.525) ccw
  line L86 (44.1, 2.525) -> (32.1, 2.525)
  arc A78 (31.1, 3.525) -> (32.1, 2.525) centre (32.1, 3.525) ccw
  line L87 (31.1, 3.525) -> (31.1, 15.525)
  arc A79 (32.1, 16.525) -> (31.1, 15.525) centre (32.1, 15.525) ccw
  line L88 (32.1, 16.525) -> (44.1, 16.525)
  arc A80 (55.9125, 35.575) -> (54.9125, 34.575) centre (55.9125, 34.575) ccw
  line L89 (55.9125, 35.575) -> (67.9125, 35.575)
  arc A81 (68.9125, 34.575) -> (67.9125, 35.575) centre (67.9125, 34.575) ccw
  line L90 (68.9125, 34.575) -> (68.9125, 22.575)
  arc A82 (67.9125, 21.575) -> (68.9125, 22.575) centre (67.9125, 22.575) ccw
  line L91 (67.9125, 21.575) -> (55.9125, 21.575)
  arc A83 (54.9125, 22.575) -> (55.9125, 21.575) centre (55.9125, 22.575) ccw
  line L92 (54.9125, 22.575) -> (54.9125, 34.575)
  arc A84 (46.3875, 54.625) -> (45.3875, 53.625) centre (46.3875, 53.625) ccw
  line L93 (46.3875, 54.625) -> (58.3875, 54.625)
  arc A85 (59.3875, 53.625) -> (58.3875, 54.625) centre (58.3875, 53.625) ccw
  line L94 (59.3875, 53.625) -> (59.3875, 41.625)
  arc A86 (58.3875, 40.625) -> (59.3875, 41.625) centre (58.3875, 41.625) ccw
  line L95 (58.3875, 40.625) -> (46.3875, 40.625)
  arc A87 (45.3875, 41.625) -> (46.3875, 40.625) centre (46.3875, 41.625) ccw
  line L96 (45.3875, 41.625) -> (45.3875, 53.625)
  arc A88 (70.2, 16.525) -> (69.2, 15.525) centre (70.2, 15.525) ccw
  line L97 (70.2, 16.525) -> (82.2, 16.525)
  arc A89 (83.2, 15.525) -> (82.2, 16.525) centre (82.2, 15.525) ccw
  line L98 (83.2, 15.525) -> (83.2, 3.525)
  arc A90 (82.2, 2.525) -> (83.2, 3.525) centre (82.2, 3.525) ccw
  line L99 (82.2, 2.525) -> (70.2, 2.525)
  arc A91 (69.2, 3.525) -> (70.2, 2.525) centre (70.2, 3.525) ccw
  line L100 (69.2, 3.525) -> (69.2, 15.525)
  arc A92 (172.5938, 73.675) -> (171.5938, 72.675) centre (172.5938, 72.675) ccw
  line L101 (172.5938, 73.675) -> (184.5938, 73.675)
  arc A93 (185.5937, 72.675) -> (184.5938, 73.675) centre (184.5937, 72.675) ccw
  line L102 (185.5937, 72.675) -> (185.5937, 60.675)
  arc A94 (184.5938, 59.675) -> (185.5937, 60.675) centre (184.5938, 60.675) ccw
  line L103 (184.5938, 59.675) -> (172.5937, 59.675)
  arc A95 (171.5938, 60.675) -> (172.5938, 59.675) centre (172.5938, 60.675) ccw
  line L104 (171.5937, 60.675) -> (171.5938, 72.675)
  arc A96 (151.1625, 35.575) -> (150.1625, 34.575) centre (151.1625, 34.575) ccw
  line L105 (151.1625, 35.575) -> (163.1625, 35.575)
  arc A97 (164.1625, 34.575) -> (163.1625, 35.575) centre (163.1625, 34.575) ccw
  line L106 (164.1625, 34.575) -> (164.1625, 22.575)
  arc A98 (163.1625, 21.575) -> (164.1625, 22.575) centre (163.1625, 22.575) ccw
  line L107 (163.1625, 21.575) -> (151.1625, 21.575)
  arc A99 (150.1625, 22.575) -> (151.1625, 21.575) centre (151.1625, 22.575) ccw
  line L108 (150.1625, 22.575) -> (150.1625, 34.575)
  arc A100 (89.25, 16.525) -> (88.25, 15.525) centre (89.25, 15.525) ccw
  line L109 (89.25, 16.525) -> (101.25, 16.525)
  arc A101 (102.25, 15.525) -> (101.25, 16.525) centre (101.25, 15.525) ccw
  line L110 (102.25, 15.525) -> (102.25, 3.525)
  arc A102 (101.25, 2.525) -> (102.25, 3.525) centre (101.25, 3.525) ccw
  line L111 (101.25, 2.525) -> (89.25, 2.525)
  arc A103 (88.25, 3.525) -> (89.25, 2.525) centre (89.25, 3.525) ccw
  line L112 (88.25, 3.525) -> (88.25, 15.525)
  arc A104 (41.625, 73.675) -> (40.625, 72.675) centre (41.625, 72.675) ccw
  line L113 (41.625, 73.675) -> (53.625, 73.675)
  arc A105 (54.625, 72.675) -> (53.625, 73.675) centre (53.625, 72.675) ccw
  line L114 (54.625, 72.675) -> (54.625, 60.675)
  arc A106 (53.625, 59.675) -> (54.625, 60.675) centre (53.625, 60.675) ccw
  line L115 (53.625, 59.675) -> (41.625, 59.675)
  arc A107 (40.625, 60.675) -> (41.625, 59.675) centre (41.625, 60.675) ccw
  line L116 (40.625, 60.675) -> (40.625, 72.675)
  arc A108 (74.9625, 35.575) -> (73.9625, 34.575) centre (74.9625, 34.575) ccw
  line L117 (74.9625, 35.575) -> (86.9625, 35.575)
  arc A109 (87.9625, 34.575) -> (86.9625, 35.575) centre (86.9625, 34.575) ccw
  line L118 (87.9625, 34.575) -> (87.9625, 22.575)
  arc A110 (86.9625, 21.575) -> (87.9625, 22.575) centre (86.9625, 22.575) ccw
  line L119 (86.9625, 21.575) -> (74.9625, 21.575)
  arc A111 (73.9625, 22.575) -> (74.9625, 21.575) centre (74.9625, 22.575) ccw
  line L120 (73.9625, 22.575) -> (73.9625, 34.575)
  arc A112 (208.3125, 35.575) -> (207.3125, 34.575) centre (208.3125, 34.575) ccw
  line L121 (208.3125, 35.575) -> (220.3125, 35.575)
  arc A113 (221.3125, 34.575) -> (220.3125, 35.575) centre (220.3125, 34.575) ccw
  line L122 (221.3125, 34.575) -> (221.3125, 22.575)
  arc A114 (220.3125, 21.575) -> (221.3125, 22.575) centre (220.3125, 22.575) ccw
  line L123 (220.3125, 21.575) -> (208.3125, 21.575)
  arc A115 (207.3125, 22.575) -> (208.3125, 21.575) centre (208.3125, 22.575) ccw
  line L124 (207.3125, 22.575) -> (207.3125, 34.575)
  arc A116 (8.2875, 16.525) -> (7.2875, 15.525) centre (8.2875, 15.525) ccw
  line L125 (8.2875, 16.525) -> (20.2875, 16.525)
  arc A117 (21.2875, 15.525) -> (20.2875, 16.525) centre (20.2875, 15.525) ccw
  line L126 (21.2875, 15.525) -> (21.2875, 3.525)
  arc A118 (20.2875, 2.525) -> (21.2875, 3.525) centre (20.2875, 3.525) ccw
  line L127 (20.2875, 2.525) -> (8.2875, 2.525)
  arc A119 (7.2875, 3.525) -> (8.2875, 2.525) centre (8.2875, 3.525) ccw
  line L128 (7.2875, 3.525) -> (7.2875, 15.525)
  arc A120 (51.15, 16.525) -> (50.15, 15.525) centre (51.15, 15.525) ccw
  line L129 (51.15, 16.525) -> (63.15, 16.525)
  arc A121 (64.15, 15.525) -> (63.15, 16.525) centre (63.15, 15.525) ccw
  line L130 (64.15, 15.525) -> (64.15, 3.525)
  arc A122 (63.15, 2.525) -> (64.15, 3.525) centre (63.15, 3.525) ccw
  line L131 (63.15, 2.525) -> (51.15, 2.525)
  arc A123 (50.15, 3.525) -> (51.15, 2.525) centre (51.15, 3.525) ccw
  line L132 (50.15, 3.525) -> (50.15, 15.525)
  arc A124 (198.7875, 54.625) -> (197.7875, 53.625) centre (198.7875, 53.625) ccw
  line L133 (198.7875, 54.625) -> (210.7875, 54.625)
  arc A125 (211.7875, 53.625) -> (210.7875, 54.625) centre (210.7875, 53.625) ccw
  line L134 (211.7875, 53.625) -> (211.7875, 41.625)
  arc A126 (210.7875, 40.625) -> (211.7875, 41.625) centre (210.7875, 41.625) ccw
  line L135 (210.7875, 40.625) -> (198.7875, 40.625)
  arc A127 (197.7875, 41.625) -> (198.7875, 40.625) centre (198.7875, 41.625) ccw
  line L136 (197.7875, 41.625) -> (197.7875, 53.625)
  arc A128 (224.9813, 73.675) -> (223.9813, 72.675) centre (224.9813, 72.675) ccw
  line L137 (224.9813, 73.675) -> (236.9813, 73.675)
  arc A129 (237.9812, 72.675) -> (236.9813, 73.675) centre (236.9813, 72.675) ccw
  line L138 (237.9812, 72.675) -> (237.9813, 60.675)
  arc A130 (236.9813, 59.675) -> (237.9813, 60.675) centre (236.9813, 60.675) ccw
  line L139 (236.9813, 59.675) -> (224.9813, 59.675)
  arc A131 (223.9812, 60.675) -> (224.9813, 59.675) centre (224.9813, 60.675) ccw
  line L140 (223.9812, 60.675) -> (223.9813, 72.675)
  arc A132 (170.2125, 35.575) -> (169.2125, 34.575) centre (170.2125, 34.575) ccw
  line L141 (170.2125, 35.575) -> (182.2125, 35.575)
  arc A133 (183.2125, 34.575) -> (182.2125, 35.575) centre (182.2125, 34.575) ccw
  line L142 (183.2125, 34.575) -> (183.2125, 22.575)
  arc A134 (182.2125, 21.575) -> (183.2125, 22.575) centre (182.2125, 22.575) ccw
  line L143 (182.2125, 21.575) -> (170.2125, 21.575)
  arc A135 (169.2125, 22.575) -> (170.2125, 21.575) centre (170.2125, 22.575) ccw
  line L144 (169.2125, 22.575) -> (169.2125, 34.575)
  arc A136 (127.35, 16.525) -> (126.35, 15.525) centre (127.35, 15.525) ccw
  line L145 (127.35, 16.525) -> (139.35, 16.525)
  arc A137 (140.35, 15.525) -> (139.35, 16.525) centre (139.35, 15.525) ccw
  line L146 (140.35, 15.525) -> (140.35, 3.525)
  arc A138 (139.35, 2.525) -> (140.35, 3.525) centre (139.35, 3.525) ccw
  line L147 (139.35, 2.525) -> (127.35, 2.525)
  arc A139 (126.35, 3.525) -> (127.35, 2.525) centre (127.35, 3.525) ccw
  line L148 (126.35, 3.525) -> (126.35, 15.525)
  arc A140 (113.0625, 35.575) -> (112.0625, 34.575) centre (113.0625, 34.575) ccw
  line L149 (113.0625, 35.575) -> (125.0625, 35.575)
  arc A141 (126.0625, 34.575) -> (125.0625, 35.575) centre (125.0625, 34.575) ccw
  line L150 (126.0625, 34.575) -> (126.0625, 22.575)
  arc A142 (125.0625, 21.575) -> (126.0625, 22.575) centre (125.0625, 22.575) ccw
  line L151 (125.0625, 21.575) -> (113.0625, 21.575)
  arc A143 (112.0625, 22.575) -> (113.0625, 21.575) centre (113.0625, 22.575) ccw
  line L152 (112.0625, 22.575) -> (112.0625, 34.575)
  arc A144 (146.4, 16.525) -> (145.4, 15.525) centre (146.4, 15.525) ccw
  line L153 (146.4, 16.525) -> (158.4, 16.525)
  arc A145 (159.4, 15.525) -> (158.4, 16.525) centre (158.4, 15.525) ccw
  line L154 (159.4, 15.525) -> (159.4, 3.525)
  arc A146 (158.4, 2.525) -> (159.4, 3.525) centre (158.4, 3.525) ccw
  line L155 (158.4, 2.525) -> (146.4, 2.525)
  arc A147 (145.4, 3.525) -> (146.4, 2.525) centre (146.4, 3.525) ccw
  line L156 (145.4, 3.525) -> (145.4, 15.525)
  arc A148 (189.2625, 35.575) -> (188.2625, 34.575) centre (189.2625, 34.575) ccw
  line L157 (189.2625, 35.575) -> (201.2625, 35.575)
  arc A149 (202.2625, 34.575) -> (201.2625, 35.575) centre (201.2625, 34.575) ccw
  line L158 (202.2625, 34.575) -> (202.2625, 22.575)
  arc A150 (201.2625, 21.575) -> (202.2625, 22.575) centre (201.2625, 22.575) ccw
  line L159 (201.2625, 21.575) -> (189.2625, 21.575)
  arc A151 (188.2625, 22.575) -> (189.2625, 21.575) centre (189.2625, 22.575) ccw
  line L160 (188.2625, 22.575) -> (188.2625, 34.575)
  arc A152 (203.55, 16.525) -> (202.55, 15.525) centre (203.55, 15.525) ccw
  line L161 (203.55, 16.525) -> (215.55, 16.525)
  arc A153 (216.55, 15.525) -> (215.55, 16.525) centre (215.55, 15.525) ccw
  line L162 (216.55, 15.525) -> (216.55, 3.525)
  arc A154 (215.55, 2.525) -> (216.55, 3.525) centre (215.55, 3.525) ccw
  line L163 (215.55, 2.525) -> (203.55, 2.525)
  arc A155 (202.55, 3.525) -> (203.55, 2.525) centre (203.55, 3.525) ccw
  line L164 (202.55, 3.525) -> (202.55, 15.525)
  arc A156 (108.3, 16.525) -> (107.3, 15.525) centre (108.3, 15.525) ccw
  line L165 (108.3, 16.525) -> (120.3, 16.525)
  arc A157 (121.3, 15.525) -> (120.3, 16.525) centre (120.3, 15.525) ccw
  line L166 (121.3, 15.525) -> (121.3, 3.525)
  arc A158 (120.3, 2.525) -> (121.3, 3.525) centre (120.3, 3.525) ccw
  line L167 (120.3, 2.525) -> (108.3, 2.525)
  arc A159 (107.3, 3.525) -> (108.3, 2.525) centre (108.3, 3.525) ccw